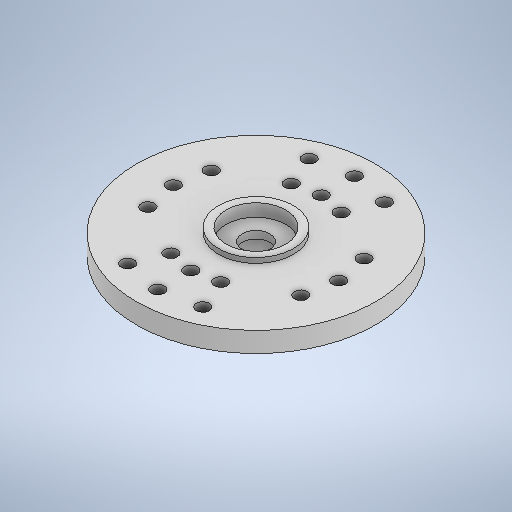
# Autodesk Inventor part: MMAE 232 Assignment 2_White Circle - Dylan Tamras
Saved by Autodesk Inventor 2025.2 (Build 292293000, 293)
## iProperties
Created: 2025-01-19
Part Number: MMAE 232 Assignment 2_White Circle - Dylan Tamras
Material: Generic
Document SubType Name: Modeling
Designer: Dylan
Density: 1 g/cm^3
Appearance: Default
Author: Dylan
Autodesk Inventor part; units mm, degrees
ref_plane "YZ Plane" through (0, 0, 0) normal (1, 0, 0) x (0, 1, 0)
ref_plane "XZ Plane" through (0, 0, 0) normal (0, 1, 0) x (-1, 0, 0)
ref_plane "XY Plane" through (0, 0, 0) normal (0, 0, 1) x (1, 0, 0)
sketch "Sketch1" plane through (0, 0, 0) normal (0, 1, 0) x (-1, 0, 0)
  circle A0 centre (0, 0) radius 11.915
  dimension "d0" = 23.83
  constraints: 1 centre point, 1 coincident
  measures "d0" diameter of A0
extrude "Extrusion1" add sketch "Sketch1" along normal blind 2
sketch "Sketch2" plane through (0, 2, 0) normal (0, 1, 0) x (1, 0, 0)
  circle A0 centre (0, 6.5) radius 0.65
  line L0 (0, 0) -> (6.5, 0) construction
  circle A1 centre (2.4874, 6.0052) radius 0.65
  circle A2 centre (8.25, 0) radius 0.65
  line L1 (0, 0) -> (8.25, 0) construction
  circle A3 centre (7.622, 3.1571) radius 0.65
  circle A4 centre (0, 9.8) radius 0.65
  line L2 (0, 0) -> (9.8, 0) construction
  circle A5 centre (3.7503, 9.054) radius 0.65
  circle A6 centre (0, 0) radius 11.915 projected
  circle A7 centre (-2.4874, 6.0052) radius 0.65
  circle A8 centre (-8.25, 0) radius 0.65
  circle A9 centre (-7.622, 3.1571) radius 0.65
  circle A10 centre (-3.7503, 9.054) radius 0.65
  circle A11 centre (0, -6.5) radius 0.65
  circle A12 centre (2.4874, -6.0052) radius 0.65
  circle A13 centre (7.622, -3.1571) radius 0.65
  circle A14 centre (0, -9.8) radius 0.65
  circle A15 centre (3.7503, -9.054) radius 0.65
  circle A16 centre (-3.7503, -9.054) radius 0.65
  circle A17 centre (-2.4874, -6.0052) radius 0.65
  circle A18 centre (-7.622, -3.1571) radius 0.65
  dimension "d5" = 1.3
  dimension "d8" = 1.3
  dimension "d10" = 1.3
  dimension "d13" = 1.3
  dimension "d15" = 1.3
  dimension "d18" = 1.3
  constraints: 18 centre point, 6 end point, 3 coincident, 3 horizontal
  measures "d5" diameter of A0
  measures "d8" diameter of A1
  measures "d10" diameter of A2
  measures "d13" diameter of A3
  measures "d15" diameter of A4
  measures "d18" diameter of A5
extrude "Extrusion2" cut sketch "Sketch2" against normal blind 2 contours A0 | A1 | A2 | A3 | A4 | A5 | A7 | A8 | A9 | A10 | A11 | A12 | A13 | A14 | A15 | A16 | A17 | A18
sketch "Sketch3" plane through (0, 2, 0) normal (0, 1, 0) x (1, 0, 0)
  circle A0 centre (0, 0) radius 3.73
  dimension "d21" = 7.46
  constraints: 1 centre point, 1 coincident
  measures "d21" diameter of A0
extrude "Extrusion3" add sketch "Sketch3" along normal blind 0.5
sketch "Sketch4" plane through (0, 2.5, 0) normal (0, 1, 0) x (1, 0, 0)
  circle A0 centre (0, 0) radius 2.97
  dimension "d24" = 5.94
  constraints: 1 centre point, 1 coincident
  measures "d24" diameter of A0
extrude "Extrusion4" cut sketch "Sketch4" against normal blind 1.25
sketch "Sketch5" plane through (0, 1.25, 0) normal (0, 1, 0) x (1, 0, 0)
  circle A0 centre (0, 0) radius 1.37
  dimension "d27" = 2.74
  constraints: 1 centre point, 1 coincident
  measures "d27" diameter of A0
extrude "Extrusion5" cut sketch "Sketch5" against normal blind 0.75
sketch "Sketch6" plane through (0, 0, 0) normal (0, -1, 0) x (1, 0, 0)
  circle A0 centre (0, 0) radius 4.44
  dimension "d30" = 8.88
  constraints: 1 centre point, 1 coincident
  measures "d30" diameter of A0
extrude "Extrusion6" add sketch "Sketch6" along normal blind 2.5
sketch "Sketch7" plane through (0, -2.5, 0) normal (0, -1, 0) x (1, 0, 0)
  circle A0 centre (0, 0) radius 2.75
  dimension "d33" = 5.5
  constraints: 1 centre point, 1 coincident
  measures "d33" diameter of A0
extrude "Extrusion7" cut sketch "Sketch7" against normal blind 3
body "Solid1"
